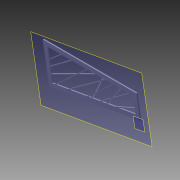
# Autodesk Inventor part: Panel_side
Saved by Autodesk Inventor 2013 (Build 170138000, 138)
## iProperties
Created: 2013-02-01
Part Number: Panel_side
Material: Aluminum 6061
Document SubType Name: Modeling
Designer: xylzlyx
Density: 1 g/cm^3
Author: xylzlyx
Autodesk Inventor part; units mm, degrees
ref_plane "YZ Plane" through (0, 0, 0) normal (1, 0, 0) x (0, 1, 0)
ref_plane "XZ Plane" through (0, 0, 0) normal (0, 1, 0) x (-1, 0, 0)
ref_plane "XY Plane" through (0, 0, 0) normal (0, 0, 1) x (1, 0, 0)
ref_plane "Work Plane2" through (0, 0, -10) normal (0, 0, -1) x (-0.9848078, -0.1736482, 0)
ref_plane "Work Plane1" through (0, 0, 0) normal (0, 0, -1) x (-0.9848078, -0.1736482, 0)
sketch "Sketch1" plane through (0, 0, -10) normal (0, 0, -1) x (-0.9848078, -0.1736482, 0)
  line L0 (4, 54.6856) -> (7, 54.6856) construction
  line L1 (7, 54.6856) -> (7, 0) construction
  line L2 (7, 0) -> (4, 0) construction
  line L3 (4, 0) -> (4, 54.6856) construction
  line L4 (246.7229, -3) -> (0, -3) construction
  line L5 (0, -3) -> (0, 0) construction
  line L6 (0, 0) -> (246.7229, 0) construction
  line L7 (246.7229, 0) -> (246.7229, -3) construction
  line L8 (0, 57.5265) -> (246.2019, 100.9386) construction
  line L9 (246.2019, 100.9386) -> (246.7229, 97.9842) construction
  line L10 (246.7229, 97.9842) -> (0.5209, 54.5721) construction
  line L11 (0.5209, 54.5721) -> (0, 57.5265) construction
  line L12 (242.7229, 94.2788) -> (242.7229, 0) construction
  line L13 (242.7229, 0) -> (239.7229, 0) construction
  line L14 (239.7229, 0) -> (239.7229, 94.2788) construction
  line L15 (239.7229, 94.2788) -> (242.7229, 94.2788) construction
  line L16 (239.7229, 96.7499) -> (239.7229, 0)
  line L17 (239.7229, 0) -> (7, 0)
  line L18 (7, 55.7145) -> (7, 0)
  line L19 (7, 55.7145) -> (239.7229, 96.7499)
  constraints: 40 end point, 6 horizontal, 6 vertical, 3 collinear, 2 coincident, 2 point on line, 2 vertical alignment, 1 parallel, 19 other
extrude "Extrusion1" add sketch "Sketch1" along normal blind 3
fillet "Corners" radius 1 4 edges at (-252.8814, 53.6526, -11.5) (-236.081, -41.6274, -11.5) (-6.8937, -1.2155, -11.5) (-16.5684, 53.6526, -11.5)
sketch "Sketch2" plane through (0, 0, -10) normal (0, 0, 1) x (0.9848078, 0.1736482, 0)
  line L0 (-7.8264, 55.8602) -> (-238.5492, 96.5429) projected
  line L1 (-239.7229, 95.5581) -> (-239.7229, 1) projected
  line L2 (-238.7229, 0) -> (-8, 0) projected
  line L3 (-7, 1) -> (-7, 54.8754) projected
  arc A0 (-7, 54.8754) -> (-7.8264, 55.8602) centre (-8, 54.8754) ccw construction
  line L4 (-7.8264, 55.8602) -> (-238.5492, 96.5429) construction
  arc A1 (-238.5492, 96.5429) -> (-239.7229, 95.5581) centre (-238.7229, 95.5581) ccw construction
  line L5 (-239.7229, 95.5581) -> (-239.7229, 1) construction
  arc A2 (-239.7229, 1) -> (-238.7229, 0) centre (-238.7229, 1) ccw construction
  line L6 (-238.7229, 0) -> (-8, 0) construction
  arc A3 (-8, 0) -> (-7, 1) centre (-8, 1) ccw construction
  line L7 (-7, 1) -> (-7, 54.8754) construction
  line L8 (-229.7229, 84.8323) -> (-229.7229, 10)
  line L9 (-229.7229, 10) -> (-17, 10)
  line L10 (-17, 10) -> (-17, 47.3235)
  line L11 (-17, 47.3235) -> (-229.7229, 84.8323)
  point P0 (0, 0)
  dimension "d4" = 10
  dimension "d5" = 10
  dimension "d6" = 10
  dimension "d7" = 10
  dimension "d8" = 10
  dimension "d9" = 10
  dimension "d10" = 10
  dimension "d11" = 10
  constraints: 8 end point, 1 parallel
  measures "d4" distance from line of L0 L8.start
  measures "d5" distance from line of L1 L8.start
  measures "d6" distance from line of L2 L8.end
  measures "d7" distance from line of L1 L8.end
  measures "d8" distance from line of L3 L10.end
  measures "d9" distance from line of L3 L9.end
  measures "d10" distance from line of L2 L9.end
  measures "d11" distance from line of L0 L10.end
extrude "RemoveCenter" cut sketch "Sketch2" against normal blind 3
fillet "InsideCorners" radius 1 4 edges at (-227.9694, -30.0429, -11.5) (-240.9639, 43.6526, -11.5) (-18.4782, 6.8961, -11.5) (-24.9594, 43.6526, -11.5)
sketch "Sketch3" plane through (0, 0, -10) normal (0, 0, 1) x (0.9848078, 0.1736482, 0)
  line L0 (-18, 10) -> (-228.7229, 10) projected
  line L1 (-229.7229, 11) -> (-229.7229, 83.6406) projected
  line L2 (-228.5492, 84.6254) -> (-17.8264, 47.4693) projected
  line L3 (-17, 46.4844) -> (-17, 11) projected
  line L4 (-7, 1) -> (-7, 54.8754) projected
  line L5 (-223.2605, 10) -> (-132.7526, 67.7339)
  line L6 (-189.4532, 10) -> (-87.5818, 59.769)
  line L7 (-130.3397, 10) -> (-94.844, 61.0495)
  line L8 (-103.452, 10) -> (-24.3884, 48.6263)
  line L9 (-91.5898, 10) -> (-51.1939, 53.3529)
  line L10 (-61.5388, 10) -> (-17, 20.4172)
  line L11 (-229.7229, 27.2264) -> (-108.1899, 63.4028)
  line L12 (-229.7229, 45.0853) -> (-170.9748, 74.4735)
  line L13 (-229.7229, 57.4684) -> (-193.4898, 78.4435)
  line L14 (-141.0157, 10) -> (-68.3188, 56.3724)
  line L15 (-229.7229, 59.7794) -> (-196.5498, 78.983)
  line L16 (-193.4898, 78.4435) -> (-196.5498, 78.983)
  line L17 (-229.7229, 59.7794) -> (-229.7229, 57.4684)
  line L18 (-229.7229, 42.849) -> (-167.6695, 73.8906)
  line L19 (-167.6695, 73.8906) -> (-170.9748, 74.4735)
  line L20 (-229.7229, 45.0853) -> (-229.7229, 42.849)
  line L21 (-229.7229, 29.3132) -> (-112.5923, 64.179)
  line L22 (-112.5923, 64.179) -> (-108.1899, 63.4028)
  line L23 (-229.7229, 29.3132) -> (-229.7229, 27.2264)
  line L24 (-219.5416, 10) -> (-129.8391, 67.2201)
  line L25 (-129.8391, 67.2201) -> (-132.7526, 67.7339)
  line L26 (-223.2605, 10) -> (-219.5416, 10)
  line L27 (-184.897, 10) -> (-84.2339, 59.1787)
  line L28 (-87.5818, 59.769) -> (-84.2339, 59.1787)
  line L29 (-189.4532, 10) -> (-184.897, 10)
  line L30 (-137.2968, 10) -> (-65.4053, 55.8587)
  line L31 (-65.4053, 55.8587) -> (-68.3188, 56.3724)
  line L32 (-141.0157, 10) -> (-137.2968, 10)
  line L33 (-127.9038, 10) -> (-92.6741, 60.6669)
  line L34 (-92.6741, 60.6669) -> (-94.844, 61.0495)
  line L35 (-130.3397, 10) -> (-127.9038, 10)
  line L36 (-108.0082, 10) -> (-27.7363, 49.2166)
  line L37 (-108.0082, 10) -> (-103.452, 10)
  line L38 (-27.7363, 49.2166) -> (-24.3884, 48.6263)
  line L39 (-88.8561, 10) -> (-48.846, 52.9389)
  line L40 (-51.1939, 53.3529) -> (-48.846, 52.9389)
  line L41 (-88.8561, 10) -> (-91.5898, 10)
  line L42 (-70.3206, 10) -> (-17, 22.4712)
  line L43 (-70.3206, 10) -> (-61.5388, 10)
  line L44 (-17, 20.4172) -> (-17, 22.4712)
  point P0 (0, 0)
  dimension "d15" = 2
  dimension "d16" = 23.8612
  dimension "d17" = 31.9995
  dimension "d18" = 38.5553
  dimension "d19" = 57.5744
  dimension "d20" = 2
  dimension "d21" = 115.9569
  dimension "d22" = 54.3274
  dimension "d23" = 2
  dimension "d24" = 5.4623
  dimension "d25" = 95.7966
  dimension "d26" = 2
  dimension "d27" = 39.2697
  dimension "d28" = 140.9675
  dimension "d29" = 2
  dimension "d30" = 87.7071
  dimension "d31" = 160.2304
  dimension "d32" = 2
  dimension "d33" = 98.3831
  dimension "d34" = 133.7052
  dimension "d35" = 2
  dimension "d36" = 204.1608
  dimension "d37" = 125.2709
  dimension "d38" = 2
  dimension "d39" = 137.1331
  dimension "d40" = 177.3553
  dimension "d41" = 2
  dimension "d42" = 167.1841
  dimension "d43" = 26.0672
  dimension "d44" = 2
  constraints: 80 end point, 13 parallel, 8 point on line, 7 horizontal, 4 collinear, 42 other
  measures "d15" distance between parallel lines of L13 L15
  measures "d16" distance of L1.end L15.start
  measures "d17" horizontal distance of L15.end point (-228.549, 84.625)
  measures "d18" distance of L1.end L12.start
  measures "d19" horizontal distance of point (-228.549, 84.625) L12.end
  measures "d20" distance between parallel lines of L18 L12
  measures "d21" horizontal distance of point (-228.549, 84.625) L21.end
  measures "d22" distance of L1.end L21.start
  measures "d23" distance between parallel lines of L21 L11
  measures "d24" distance of point (-228.723, 10) L5.start
  measures "d25" horizontal distance of point (-228.549, 84.625) L5.end
  measures "d26" distance between parallel lines of L5 L24
  measures "d27" distance of point (-228.723, 10) L6.start
  measures "d28" horizontal distance of point (-228.549, 84.625) L6.end
  measures "d29" distance between parallel lines of L27 L6
  measures "d30" distance of point (-228.723, 10) L14.start
  measures "d31" horizontal distance of point (-228.549, 84.625) L14.end
  measures "d32" distance between parallel lines of L30 L14
  measures "d33" distance of point (-228.723, 10) L7.start
  measures "d34" horizontal distance of point (-228.549, 84.625) L7.end
  measures "d35" distance between parallel lines of L7 L33
  measures "d36" horizontal distance of point (-228.549, 84.625) L8.end
  measures "d37" distance of point (-228.723, 10) L8.start
  measures "d38" distance between parallel lines of L8 L36
  measures "d39" distance of point (-228.723, 10) L9.start
  measures "d40" horizontal distance of point (-228.549, 84.625) L9.end
  measures "d41" distance between parallel lines of L9 L39
  measures "d42" distance of point (-228.723, 10) L10.start
  measures "d43" distance of L3.start L10.end
  measures "d44" distance between parallel lines of L10 L42
extrude "Lateral" add sketch "Sketch3" against normal blind 3 contours L0 L42 L3 L10 | L0 L9 L8 L39 | L39 L36 L2 L8 | L8 L9 L36 L39 | L0 L36 L9 L8 | L36 L9 L2 L39 | L0 L7 L30 L33 | L33 L14 L2 L30 | L30 L7 L14 L33 | L0 L14 L7 L30 | L14 L7 L27 L33 | L33 L6 L2 L27 | L27 L7 L6 L33 | L0 L6 L7 L27 | L6 L7 L2 L33 | L0 L5 L11 L24 | L24 L21 L2 L11 | L11 L5 L21 L24 | L11 L1 L21 L5 | L21 L5 L2 L24 | L18 L1 L12 L2 | L13 L1 L15 L2
body "Solid1"
